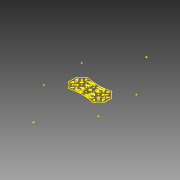
# Autodesk Inventor part: Centerplate
Saved by Autodesk Inventor 2012 (Build 160160000, 160)
## iProperties
Created: 2014-07-01
Part Number: Centerplate
Material: Default
Document SubType Name: Modeling
Designer: Laurent
Density: 1 g/cm^3
Author: Laurent
Autodesk Inventor part; units mm, degrees
ref_plane "YZ Plane" through (0, 0, 0) normal (1, 0, 0) x (0, 1, 0)
ref_plane "XZ Plane" through (0, 0, 0) normal (0, 1, 0) x (-1, 0, 0)
ref_plane "XY Plane" through (0, 0, 0) normal (0, 0, 1) x (1, 0, 0)
sketch "Sketch1" plane through (0, 0, 0) normal (0, 0, 1) x (1, 0, 0)
  line L0 (-75, 40) -> (75, 40)
  line L1 (75, 40) -> (75, -40)
  line L2 (75, -40) -> (-75, -40)
  line L3 (-75, -40) -> (-75, 40)
  point P0 (0, 0)
  dimension "d0" = 150
  dimension "d1" = 80
  dimension "d2" = 40
  dimension "d3" = 75
  constraints: 8 end point, 2 parallel, 1 horizontal, 1 perpendicular
  measures "d0" distance of L1.end L2.end
  measures "d1" distance of L0.end L1.end
  measures "d2" distance from line of L0 point (0, 0)
  measures "d3" distance from line of L1 point (0, 0)
extrude "Vlak" add sketch "Sketch1" along normal blind 4
sketch "Sketch3" plane through (0, 0, 4) normal (0, 0, 1) x (1, 0, 0)
  line L0 (75, 40) -> (75, -40) projected
  line L1 (-75, 40) -> (75, 40) projected
  circle A0 centre (75, 40) radius 10
  point P0 (0, 0)
  dimension "d12" = 20
  dimension "d13" = 0
  dimension "d14" = 0
  constraints: 1 centre point
  measures "d12" diameter of A0
  measures "d13" distance from line of L0 A0.centre
  measures "d14" distance from line of L1 A0.centre
extrude "Centergat" cut sketch "Sketch3" against normal blind 4
sketch "Sketch4" plane through (0, 0, 4) normal (0, 0, 1) x (1, 0, 0)
  line L0 (-75, 40) -> (65, 40) projected
  line L1 (75, -40) -> (-75, -40) projected
  line L2 (18.8539, 53.8539) -> (-131.8943, -96.8943) construction
  circle A0 centre (-155, -120) radius 150
  point P0 (0, 0)
  dimension "d17" = 0
  dimension "d18" = 45
  dimension "d19" = 300
  dimension "d20" = 0
  dimension "d21" = 160
  constraints: 2 end point, 1 centre point
  measures "d17" distance from line of L1.end L2
  measures "d18" angle of L1 L2
  measures "d19" diameter of A0
  measures "d20" distance from line of L2 A0.centre
  measures "d21" distance from line of L0 A0.centre
extrude "PropellorSpace" cut sketch "Sketch4" against normal blind 4
sketch "Sketch5" plane through (0, 0, 4) normal (0, 0, 1) x (1, 0, 0)
  arc A0 (-28.1142, -40) -> (-75, 6.8858) centre (-155, -120) ccw projected
  line L0 (75, -40) -> (-28.1142, -40) projected
  line L1 (-75, 40) -> (65, 40) projected
  line L2 (-155, -120) -> (34.1296, 69.1296) construction
  line L3 (-168.3606, -98.0053) -> (-8.8118, 61.5435) construction
  line L4 (-132.6124, -132.9677) -> (63.849, 63.4937) construction
  line L5 (-208.1378, -57.7825) -> (-104.1378, -161.7825) construction
  line L6 (-25.5995, -23.1264) -> (-11.4573, -8.9842)
  line L7 (-11.4573, -8.9842) -> (-8.6289, -11.8127)
  line L8 (-8.6289, -11.8127) -> (-22.771, -25.9548)
  line L9 (-22.771, -25.9548) -> (-25.5995, -23.1264)
  line L10 (-60.9548, 12.229) -> (-46.8127, 26.3711)
  line L11 (-46.8127, 26.3711) -> (-43.9842, 23.5427)
  line L12 (-43.9842, 23.5427) -> (-58.1264, 9.4005)
  line L13 (-58.1264, 9.4005) -> (-60.9548, 12.229)
  line L14 (13.2914, 15.7645) -> (27.4335, 29.9066)
  line L15 (27.4335, 29.9066) -> (30.262, 27.0782)
  line L16 (30.262, 27.0782) -> (16.1198, 12.9361)
  line L17 (16.1198, 12.9361) -> (13.2914, 15.7645)
  line L18 (-62.0184, 71.663) -> (40.1093, -30.4647) construction
  line L19 (-7.9217, 14.7379) -> (-22.0638, 28.88)
  line L20 (-22.0638, 28.88) -> (-19.2354, 31.7085)
  line L21 (-19.2354, 31.7085) -> (-5.0932, 17.5663)
  line L22 (-5.0932, 17.5663) -> (-7.9217, 14.7379)
  point P0 (0, 0)
  point P1 (-168.1378, -97.7825)
  point P2 (-132.7825, -133.1378)
  point P3 (-30.3553, 40)
  dimension "d24" = 45
  dimension "d25" = 0
  dimension "d26" = 90
  dimension "d27" = 25
  dimension "d28" = 25
  dimension "d29" = 0
  dimension "d30" = 0
  dimension "d31" = 0
  dimension "d32" = 20
  dimension "d33" = 4
  dimension "d34" = 20
  dimension "d35" = 4
  dimension "d36" = 0
  dimension "d37" = 2
  dimension "d38" = 0
  dimension "d39" = 2
  dimension "d40" = 160
  dimension "d41" = 160
  dimension "d44" = 55
  dimension "d49" = 45
  dimension "d50" = 0
  dimension "d51" = 0
  dimension "d52" = 0
  dimension "d53" = 21.2742
  dimension "d54" = 20
  dimension "d55" = 4
  dimension "d56" = 0
  dimension "d57" = 2
  dimension "d58" = 13.726
  constraints: 42 end point, 6 parallel, 4 perpendicular, 2 point on line, 1 collinear, 8 other
  measures "d24" angle of L0 L2
  measures "d25" angle of L3 L2
  measures "d26" angle of L2 L5
  measures "d27" distance from line of L2 point (-168.138, -97.783)
  measures "d28" distance from line of L2 point (-132.783, -133.138)
  measures "d29" distance from line of point (-132.783, -133.138) L4
  measures "d30" distance from line of point (-168.138, -97.783) L3
  measures "d31" angle of L4 L2
  measures "d32" distance of L7.end L8.end
  measures "d33" distance of L6.end L7.end
  measures "d34" distance of L11.end L13.start
  measures "d35" distance of L10.end L11.end
  measures "d36" angle of L3 L10
  measures "d37" distance from line of L3 L10.end
  measures "d38" angle of L4 L6
  measures "d39" distance from line of L4 L7.end
  measures "d40" distance from line of L2.start L13
  measures "d41" distance from line of L2.start L9
  measures "d44" distance of L7.end L16.start
  measures "d49" angle of L1 L18
  measures "d50" distance from line of L3 point (-30.355, 40)
  measures "d51" distance from line of L1 point (-30.355, 40)
  measures "d52" distance from line of point (-30.355, 40) L18
  measures "d53" distance from line of point (-30.355, 40) L11
  measures "d54" distance of L20.end L21.end
  measures "d55" distance of L19.end L20.end
  measures "d56" angle of L18 L19
  measures "d57" distance from line of L18 L20.end
  measures "d58" distance from line of L20 point (-30.355, 40)
extrude "Armsteunen" cut sketch "Sketch5" against normal blind 4
sketch "Sketch6" plane through (0, 0, 4) normal (0, 0, 1) x (1, 0, 0)
  line L0 (75, -40) -> (-28.1142, -40) projected
  line L1 (75, 30) -> (75, -40) projected
  line L2 (-75, 40) -> (65, 40) projected
  line L3 (-75, 6.8858) -> (-75, 40) projected
  circle A0 centre (55, -20) radius 1.5
  circle A1 centre (15, -20) radius 1.5
  circle A2 centre (-13.9878, -20) radius 1.5
  circle A3 centre (-34.4939, 0.5061) radius 1.5
  circle A4 centre (43.89, 40) radius 1.5
  circle A5 centre (26.0122, 20) radius 1.5
  circle A6 centre (5, 40) radius 1.5
  circle A7 centre (-55, 21.0122) radius 1.5
  circle A8 centre (-55, 30) radius 1.5
  line L4 (-55, 21.0122) -> (-13.9878, -20) construction
  line L5 (-34.4939, 0.5061) -> (12.7873, 47.7873) construction
  circle A9 centre (-40.4428, 35) radius 1.5
  circle A10 centre (3.6899, -2.3223) radius 1.5
  circle A11 centre (-16.8162, 18.1838) radius 1.5
  arc A12 (65, 40) -> (75, 30) centre (75, 40) ccw projected
  circle A13 centre (75, 8.89) radius 1.5
  point P0 (0, 0)
  point P1 (-43.9842, 23.5427)
  point P2 (-11.4573, -8.9842)
  dimension "d61" = 3
  dimension "d62" = 3
  dimension "d63" = 3
  dimension "d64" = 3
  dimension "d65" = 3
  dimension "d66" = 3
  dimension "d67" = 3
  dimension "d68" = 3
  dimension "d69" = 3
  dimension "d70" = 20
  dimension "d71" = 20
  dimension "d72" = 20
  dimension "d73" = 60
  dimension "d75" = 20
  dimension "d76" = 31.11
  dimension "d77" = 0
  dimension "d78" = 20
  dimension "d80" = 10
  dimension "d82" = 20
  dimension "d83" = 20
  dimension "d84" = 0
  dimension "d87" = 45
  dimension "d88" = 0
  dimension "d89" = 0
  dimension "d90" = 3
  dimension "d101" = 3
  dimension "d103" = 29
  dimension "d106" = 3
  dimension "d107" = 0
  dimension "d111" = 3
  dimension "d112" = 0
  dimension "d113" = 31.11
  dimension "d166" = 29
  dimension "d167" = 23
  dimension "d168" = 23
  dimension "d169" = 29
  dimension "d170" = 25
  dimension "d171" = 25
  dimension "d172" = 29
  dimension "d175" = 29
  dimension "d179" = 5
  dimension "d182" = 43.9962
  constraints: 13 centre point, 4 end point
  measures "d61" diameter of A0
  measures "d62" diameter of A1
  measures "d63" diameter of A2
  measures "d64" diameter of A3
  measures "d65" diameter of A4
  measures "d66" diameter of A5
  measures "d67" diameter of A6
  measures "d68" diameter of A7
  measures "d69" diameter of A8
  measures "d70" distance from line of L1 A0.centre
  measures "d71" distance from line of L0 A0.centre
  measures "d72" distance from line of L0 A1.centre
  measures "d73" distance from line of L1 A1.centre
  measures "d75" distance from line of L0 L4.end
  measures "d76" distance from line of L1 A4.centre
  measures "d77" distance from line of L2 A4.centre
  measures "d78" distance from line of L2 A5.centre
  measures "d80" distance from line of L2 A8.centre
  measures "d82" distance from line of L3 L4.start
  measures "d83" distance from line of L3 A8.centre
  measures "d84" distance from line of L4 L5.start
  measures "d87" angle of L2 L5
  measures "d88" distance from line of L2 A6.centre
  measures "d89" distance from line of L5 A6.centre
  measures "d90" diameter of A9
  measures "d101" diameter of A10
  measures "d103" distance from line of A10.centre L5
  measures "d106" diameter of A11
  measures "d107" distance from line of L5 A11.centre
  measures "d111" diameter of A13
  measures "d112" distance from line of L1 A13.centre
  measures "d113" distance of A12.centre A13.centre
  measures "d166" distance from line of L4.end L5
  measures "d167" distance from line of point (-11.457, -8.984) L5
  measures "d168" distance from line of point (-43.984, 23.543) L5
  measures "d169" distance from line of L4.start L5
  measures "d170" distance of A11.centre L5.start
  measures "d171" distance of A10.centre L4.end
  measures "d172" distance of A9.centre A11.centre
  measures "d175" distance from line of L5 A5.centre
  measures "d179" distance from line of A9.centre L2
  measures "d182" distance of A13.centre A4.centre
extrude "Holes" cut sketch "Sketch6" against normal blind 4
sketch "Sketch10" plane through (0, 0, 4) normal (0, 0, 1) x (1, 0, 0)
  line L0 (45.39, 40) -> (65, 40) projected
  line L1 (6.5, 40) -> (42.39, 40) projected
  line L2 (75, 7.39) -> (75, -40) projected
  line L3 (45, -8) -> (65, -8)
  line L4 (65, -8) -> (65, -12)
  line L5 (65, -12) -> (45, -12)
  line L6 (45, -12) -> (45, -8)
  line L7 (31, 30) -> (35, 30)
  line L8 (35, 30) -> (35, 10)
  line L9 (35, 10) -> (31, 10)
  line L10 (31, 10) -> (31, 30)
  line L11 (5, -8) -> (25, -8)
  line L12 (25, -8) -> (25, -12)
  line L13 (25, -12) -> (5, -12)
  line L14 (5, -12) -> (5, -8)
  point P0 (0, 0)
  point P1 (-8.6289, -11.8127)
  dimension "d114" = 20
  dimension "d115" = 4
  dimension "d116" = 4
  dimension "d117" = 20
  dimension "d118" = 10
  dimension "d119" = 48
  dimension "d120" = 40
  dimension "d121" = 10
  dimension "d124" = 40
  dimension "d164" = 13.6289
  dimension "d165" = 10
  constraints: 24 end point, 4 parallel, 3 horizontal, 2 perpendicular, 1 collinear, 7 other
  measures "d114" distance of L4.end L5.end
  measures "d115" distance of L3.end L4.end
  measures "d116" distance of L8.end L9.end
  measures "d117" distance of L7.end L8.end
  measures "d118" distance from line of L2 L4.end
  measures "d119" distance between parallel lines of L0 L3
  measures "d120" distance between parallel lines of L2 L8
  measures "d121" distance between parallel lines of L1 L7
  measures "d124" distance of L3.start L14.end
  measures "d164" distance from line of L14 point (-8.629, -11.813)
  measures "d165" distance between parallel lines of L6 L8
extrude "InternalStructure" cut sketch "Sketch10" against normal blind 4
sketch "Sketch11" plane through (0, 0, 4) normal (0, 0, 1) x (1, 0, 0)
  line L0 (25, -8) -> (25, -12) projected
  line L1 (-25.5995, -23.1264) -> (-11.4573, -8.9842) projected
  circle A0 centre (15, -20) radius 1.5 projected
  circle A1 centre (-34.4939, 0.5061) radius 1.5 projected
  line L2 (6.5, 40) -> (42.39, 40) projected
  line L3 (75, 7.39) -> (75, -40) projected
  line L4 (40, 25) -> (50, 25)
  line L5 (50, 25) -> (50, 0)
  line L6 (50, 0) -> (40, 0)
  line L7 (40, 0) -> (40, 25)
  line L8 (25, -15) -> (45, -15)
  line L9 (45, -15) -> (45, -25)
  line L10 (45, -25) -> (25, -25)
  line L11 (25, -25) -> (25, -15)
  line L12 (-24.6985, 17.3726) -> (-17.6274, 10.3015)
  line L13 (-17.6274, 10.3015) -> (-28.234, -0.3051)
  line L14 (-28.234, -0.3051) -> (-35.3051, 6.766)
  line L15 (-35.3051, 6.766) -> (-24.6985, 17.3726)
  line L16 (-7.9217, 14.7379) -> (-22.0638, 28.88) projected
  point P0 (0, 0)
  dimension "d134" = 10
  dimension "d135" = 25
  dimension "d136" = 25
  dimension "d137" = 15
  dimension "d138" = 20
  dimension "d139" = 10
  dimension "d140" = 0
  dimension "d141" = 5
  dimension "d142" = 10
  dimension "d144" = 0
  dimension "d145" = 5
  dimension "d180" = 10
  dimension "d181" = 15
  constraints: 24 end point, 6 parallel, 3 perpendicular, 2 horizontal
  measures "d134" distance of L5.end L6.end
  measures "d135" distance of L4.end L5.end
  measures "d136" distance between parallel lines of L3 L5
  measures "d137" distance between parallel lines of L2 L4
  measures "d138" distance of L9.end L10.end
  measures "d139" distance of L8.end L9.end
  measures "d140" distance between parallel lines of L0 L11
  measures "d141" distance from line of L8 A0.centre
  measures "d142" distance of L13.end L14.end
  measures "d144" angle of L1 L13
  measures "d145" distance from line of A1.centre L13
  measures "d180" distance from line of L16 L12.start
  measures "d181" distance between parallel lines of L12 L14
extrude "CablingHoles" cut sketch "Sketch11" against normal blind 4 contours L4 L5 L6 L7 | L8 L9 L10 L11 | L12 L13 L14 L15
sketch "Sketch12" plane through (0, 0, 4) normal (0, 0, 1) x (1, 0, 0)
  line L0 (75, -40) -> (-28.1142, -40) projected
  line L1 (75, 7.39) -> (75, -40) projected
  arc A0 (75, -26.5) -> (-28.1142, -40) centre (76.1332, -435.7032) ccw
  line L2 (45, -25) -> (25, -25) projected
  line L3 (5, -8) -> (25, -8) projected
  line L4 (35, 30) -> (35, -49) construction
  line L5 (65, -8) -> (-10, -8) construction
  circle A1 centre (29, -5) radius 1.5
  circle A2 centre (38, -5) radius 1.5
  line L6 (16.1198, 12.9361) -> (13.2914, 15.7645) projected
  line L7 (-7.9217, 14.7379) -> (-22.0638, 28.88) projected
  line L8 (-22.0638, 28.88) -> (-19.2354, 31.7085) projected
  line L9 (-19.2354, 31.7085) -> (-5.0932, 17.5663) projected
  line L10 (-46.8127, 26.3711) -> (-43.9842, 23.5427) projected
  line L11 (-43.9842, 23.5427) -> (-58.1264, 9.4005) projected
  point P0 (0, 0)
  dimension "d149" = 13.5
  dimension "d150" = 103.1142
  dimension "d151" = 40
  dimension "d156" = 3
  dimension "d157" = 3
  dimension "d158" = 3
  dimension "d159" = 3
  dimension "d160" = 6
  dimension "d161" = 3
  dimension "d176" = 11.7258
  dimension "d177" = 11.726
  dimension "d178" = 19.2742
  constraints: 4 end point, 3 centre point, 2 point on circle, 2 point on line, 1 perpendicular
  measures "d149" distance of L0.start A0.start
  measures "d150" distance from line of L1 L0.end
  measures "d151" vertical distance of point (0, 0) L0.end
  measures "d156" diameter of A1
  measures "d157" diameter of A2
  measures "d158" distance from line of L5 A2.centre
  measures "d159" distance from line of L4 A2.centre
  measures "d160" distance from line of L4 A1.centre
  measures "d161" distance from line of L5 A1.centre
  measures "d176" distance between parallel lines of L6 L9
  measures "d177" distance between parallel lines of L8 L11
  measures "d178" distance between parallel lines of L7 L10
extrude "BodyReshape" cut sketch "Sketch12" against normal blind 4
sketch "Sketch14" plane through (0, 0, 4) normal (0, 0, 1) x (1, 0, 0)
  arc A0 (75, -26.5) -> (-28.1142, -40) centre (76.1332, -435.7032) ccw projected
  line L0 (75, 7.39) -> (75, -26.5) projected
  arc A1 (75, 10.39) -> (75, 7.39) centre (75, 8.89) ccw projected
  line L1 (75, 30) -> (75, 10.39) projected
  arc A2 (65, 40) -> (75, 30) centre (75, 40) ccw projected
  line L2 (45.39, 40) -> (65, 40) projected
  arc A3 (42.39, 40) -> (45.39, 40) centre (43.89, 40) ccw projected
  line L3 (6.5, 40) -> (42.39, 40) projected
  arc A4 (3.5, 40) -> (6.5, 40) centre (5, 40) ccw projected
  line L4 (-75, 40) -> (3.5, 40) projected
  arc A5 (-28.1142, -40) -> (-75, 6.8858) centre (-155, -120) ccw projected
  circle A6 centre (-55, 21.0122) radius 1.5 projected
  circle A7 centre (-34.4939, 0.5061) radius 1.5 projected
  circle A8 centre (-13.9878, -20) radius 1.5 projected
  circle A9 centre (55, -20) radius 1.5 projected
  circle A10 centre (-16.8162, 18.1838) radius 1.5 projected
  circle A11 centre (3.6899, -2.3223) radius 1.5 projected
  circle A12 centre (-55, 30) radius 1.5 projected
  circle A13 centre (15, -20) radius 1.5 projected
  circle A14 centre (26.0122, 20) radius 1.5 projected
  circle A15 centre (-40.4428, 35) radius 1.5 projected
  circle A16 centre (29, -5) radius 1.5 projected
  circle A17 centre (38, -5) radius 1.5 projected
  arc A18 (178.1142, -40) -> (75, -26.5) centre (73.8668, -435.7032) ccw
  arc A19 (75, 7.39) -> (75, 10.39) centre (75, 8.89) ccw
  arc A20 (75, 30) -> (85, 40) centre (75, 40) ccw
  line L5 (104.61, 40) -> (85, 40)
  arc A21 (104.61, 40) -> (107.61, 40) centre (106.11, 40) ccw
  line L6 (143.5, 40) -> (107.61, 40)
  arc A22 (143.5, 40) -> (146.5, 40) centre (145, 40) ccw
  line L7 (225, 40) -> (146.5, 40)
  line L8 (225, 6.8858) -> (225, 40)
  arc A23 (225, 6.8858) -> (178.1142, -40) centre (305, -120) ccw
  circle A24 centre (205, 21.0122) radius 1.5
  circle A25 centre (184.4939, 0.5061) radius 1.5
  circle A26 centre (163.9878, -20) radius 1.5
  circle A27 centre (95, -20) radius 1.5
  circle A28 centre (166.8162, 18.1838) radius 1.5
  circle A29 centre (146.3101, -2.3223) radius 1.5
  circle A30 centre (205, 30) radius 1.5
  circle A31 centre (135, -20) radius 1.5
  circle A32 centre (123.9878, 20) radius 1.5
  circle A33 centre (190.4428, 35) radius 1.5
  line L9 (208.1264, 9.4005) -> (210.9548, 12.229)
  line L10 (210.9548, 12.229) -> (196.8127, 26.3711)
  line L11 (196.8127, 26.3711) -> (193.9842, 23.5427)
  line L12 (193.9842, 23.5427) -> (208.1264, 9.4005)
  line L13 (155.0932, 17.5663) -> (157.9217, 14.7379)
  line L14 (157.9217, 14.7379) -> (172.0638, 28.88)
  line L15 (172.0638, 28.88) -> (169.2354, 31.7085)
  line L16 (169.2354, 31.7085) -> (155.0932, 17.5663)
  line L17 (172.771, -25.9548) -> (175.5995, -23.1264)
  line L18 (175.5995, -23.1264) -> (161.4573, -8.9842)
  line L19 (161.4573, -8.9842) -> (158.6289, -11.8127)
  line L20 (158.6289, -11.8127) -> (172.771, -25.9548)
  line L21 (136.7086, 15.7645) -> (122.5665, 29.9066)
  line L22 (122.5665, 29.9066) -> (119.738, 27.0782)
  line L23 (119.738, 27.0782) -> (133.8802, 12.9361)
  line L24 (133.8802, 12.9361) -> (136.7086, 15.7645)
  line L25 (105, -12) -> (105, -8)
  line L26 (105, -8) -> (85, -8)
  line L27 (85, -8) -> (85, -12)
  line L28 (85, -12) -> (105, -12)
  line L29 (145, -12) -> (145, -8)
  line L30 (145, -8) -> (125, -8)
  line L31 (125, -8) -> (125, -12)
  line L32 (125, -12) -> (145, -12)
  line L33 (119, 10) -> (119, 30)
  line L34 (119, 30) -> (115, 30)
  line L35 (115, 30) -> (115, 10)
  line L36 (115, 10) -> (119, 10)
  line L37 (185.3051, 6.766) -> (174.6985, 17.3726)
  line L38 (174.6985, 17.3726) -> (167.6274, 10.3015)
  line L39 (167.6274, 10.3015) -> (178.234, -0.3051)
  line L40 (178.234, -0.3051) -> (185.3051, 6.766)
  line L41 (110, 0) -> (110, 25)
  line L42 (110, 25) -> (100, 25)
  line L43 (100, 25) -> (100, 0)
  line L44 (100, 0) -> (110, 0)
  line L45 (125, -25) -> (125, -15)
  line L46 (125, -15) -> (105, -15)
  line L47 (105, -15) -> (105, -25)
  line L48 (105, -25) -> (125, -25)
  circle A34 centre (121, -5) radius 1.5
  circle A35 centre (112, -5) radius 1.5
  arc A36 (-28.1142, 120) -> (75, 106.5) centre (76.1332, 515.7032) ccw
  line L49 (75, 72.61) -> (75, 106.5)
  arc A37 (75, 72.61) -> (75, 69.61) centre (75, 71.11) ccw
  line L50 (75, 50) -> (75, 69.61)
  arc A38 (75, 50) -> (65, 40) centre (75, 40) ccw
  arc A39 (45.39, 40) -> (42.39, 40) centre (43.89, 40) ccw
  arc A40 (6.5, 40) -> (3.5, 40) centre (5, 40) ccw
  line L51 (-75, 73.1142) -> (-75, 40)
  arc A41 (-75, 73.1142) -> (-28.1142, 120) centre (-155, 200) ccw
  circle A42 centre (-55, 58.9878) radius 1.5
  circle A43 centre (-34.4939, 79.4939) radius 1.5
  circle A44 centre (-13.9878, 100) radius 1.5
  circle A45 centre (55, 100) radius 1.5
  circle A46 centre (-16.8162, 61.8162) radius 1.5
  circle A47 centre (3.6899, 82.3223) radius 1.5
  circle A48 centre (-55, 50) radius 1.5
  circle A49 centre (15, 100) radius 1.5
  circle A50 centre (26.0122, 60) radius 1.5
  circle A51 centre (-40.4428, 45) radius 1.5
  line L52 (-58.1264, 70.5995) -> (-60.9548, 67.771)
  line L53 (-60.9548, 67.771) -> (-46.8127, 53.6289)
  line L54 (-46.8127, 53.6289) -> (-43.9842, 56.4573)
  line L55 (-43.9842, 56.4573) -> (-58.1264, 70.5995)
  line L56 (-5.0932, 62.4337) -> (-7.9217, 65.2621)
  line L57 (-7.9217, 65.2621) -> (-22.0638, 51.12)
  line L58 (-22.0638, 51.12) -> (-19.2354, 48.2915)
  line L59 (-19.2354, 48.2915) -> (-5.0932, 62.4337)
  line L60 (-22.771, 105.9548) -> (-25.5995, 103.1264)
  line L61 (-25.5995, 103.1264) -> (-11.4573, 88.9842)
  line L62 (-11.4573, 88.9842) -> (-8.6289, 91.8127)
  line L63 (-8.6289, 91.8127) -> (-22.771, 105.9548)
  line L64 (13.2914, 64.2355) -> (27.4335, 50.0934)
  line L65 (27.4335, 50.0934) -> (30.262, 52.9218)
  line L66 (30.262, 52.9218) -> (16.1198, 67.0639)
  line L67 (16.1198, 67.0639) -> (13.2914, 64.2355)
  line L68 (45, 92) -> (45, 88)
  line L69 (45, 88) -> (65, 88)
  line L70 (65, 88) -> (65, 92)
  line L71 (65, 92) -> (45, 92)
  line L72 (5, 92) -> (5, 88)
  line L73 (5, 88) -> (25, 88)
  line L74 (25, 88) -> (25, 92)
  line L75 (25, 92) -> (5, 92)
  line L76 (31, 70) -> (31, 50)
  line L77 (31, 50) -> (35, 50)
  line L78 (35, 50) -> (35, 70)
  line L79 (35, 70) -> (31, 70)
  line L80 (-35.3051, 73.234) -> (-24.6985, 62.6274)
  line L81 (-24.6985, 62.6274) -> (-17.6274, 69.6985)
  line L82 (-17.6274, 69.6985) -> (-28.234, 80.3051)
  line L83 (-28.234, 80.3051) -> (-35.3051, 73.234)
  line L84 (40, 80) -> (40, 55)
  line L85 (40, 55) -> (50, 55)
  line L86 (50, 55) -> (50, 80)
  line L87 (50, 80) -> (40, 80)
  line L88 (25, 105) -> (25, 95)
  line L89 (25, 95) -> (45, 95)
  line L90 (45, 95) -> (45, 105)
  line L91 (45, 105) -> (25, 105)
  circle A52 centre (29, 85) radius 1.5
  circle A53 centre (38, 85) radius 1.5
  line L92 (100, 80) -> (110, 80)
  line L93 (115, 70) -> (119, 70)
  line L94 (100, 55) -> (100, 80)
  line L95 (110, 55) -> (100, 55)
  line L96 (119, 70) -> (119, 50)
  line L97 (119, 50) -> (115, 50)
  line L98 (115, 50) -> (115, 70)
  arc A54 (75, 69.61) -> (75, 72.61) centre (75, 71.11) ccw
  arc A55 (85, 40) -> (75, 50) centre (75, 40) ccw
  line L99 (110, 80) -> (110, 55)
  line L100 (178.234, 80.3051) -> (185.3051, 73.234)
  line L101 (167.6274, 69.6985) -> (178.234, 80.3051)
  arc A56 (178.1142, 120) -> (225, 73.1142) centre (305, 200) ccw
  circle A57 centre (184.4939, 79.4939) radius 1.5
  line L102 (161.4573, 88.9842) -> (158.6289, 91.8127)
  line L103 (175.5995, 103.1264) -> (161.4573, 88.9842)
  line L104 (158.6289, 91.8127) -> (172.771, 105.9548)
  line L105 (172.771, 105.9548) -> (175.5995, 103.1264)
  circle A58 centre (163.9878, 100) radius 1.5
  line L106 (105, 88) -> (85, 88)
  line L107 (85, 88) -> (85, 92)
  line L108 (85, 92) -> (105, 92)
  circle A59 centre (95, 100) radius 1.5
  line L109 (174.6985, 62.6274) -> (167.6274, 69.6985)
  line L110 (185.3051, 73.234) -> (174.6985, 62.6274)
  circle A60 centre (166.8162, 61.8162) radius 1.5
  line L111 (208.1264, 70.5995) -> (210.9548, 67.771)
  line L112 (196.8127, 53.6289) -> (193.9842, 56.4573)
  line L113 (193.9842, 56.4573) -> (208.1264, 70.5995)
  circle A61 centre (205, 58.9878) radius 1.5
  line L114 (210.9548, 67.771) -> (196.8127, 53.6289)
  circle A62 centre (190.4428, 45) radius 1.5
  line L115 (155.0932, 62.4337) -> (157.9217, 65.2621)
  line L116 (172.0638, 51.12) -> (169.2354, 48.2915)
  line L117 (157.9217, 65.2621) -> (172.0638, 51.12)
  line L118 (169.2354, 48.2915) -> (155.0932, 62.4337)
  circle A63 centre (205, 50) radius 1.5
  line L119 (225, 73.1142) -> (225, 40)
  circle A64 centre (112, 85) radius 1.5
  line L120 (105, 92) -> (105, 88)
  circle A65 centre (121, 85) radius 1.5
  line L121 (125, 88) -> (125, 92)
  line L122 (125, 95) -> (105, 95)
  line L123 (105, 95) -> (105, 105)
  line L124 (125, 105) -> (125, 95)
  line L125 (105, 105) -> (125, 105)
  arc A66 (75, 106.5) -> (178.1142, 120) centre (73.8668, 515.7032) ccw
  arc A67 (107.61, 40) -> (104.61, 40) centre (106.11, 40) ccw
  arc A68 (146.5, 40) -> (143.5, 40) centre (145, 40) ccw
  line L126 (133.8802, 67.0639) -> (136.7086, 64.2355)
  line L127 (136.7086, 64.2355) -> (122.5665, 50.0934)
  line L128 (122.5665, 50.0934) -> (119.738, 52.9218)
  line L129 (119.738, 52.9218) -> (133.8802, 67.0639)
  circle A69 centre (123.9878, 60) radius 1.5
  line L130 (145, 92) -> (145, 88)
  line L131 (145, 88) -> (125, 88)
  line L132 (125, 92) -> (145, 92)
  circle A70 centre (135, 100) radius 1.5
  circle A71 centre (146.3101, 82.3223) radius 1.5
  point P0 (-58.1264, 9.4005)
  point P1 (-60.9548, 12.229)
  point P2 (-46.8127, 26.3711)
  point P3 (-43.9842, 23.5427)
  point P4 (-5.0932, 17.5663)
  point P5 (-7.9217, 14.7379)
  point P6 (-22.0638, 28.88)
  point P7 (-19.2354, 31.7085)
  point P8 (-22.771, -25.9548)
  point P9 (-25.5995, -23.1264)
  point P10 (-11.4573, -8.9842)
  point P11 (-8.6289, -11.8127)
  point P12 (13.2914, 15.7645)
  point P13 (27.4335, 29.9066)
  point P14 (30.262, 27.0782)
  point P15 (16.1198, 12.9361)
  point P16 (45, -12)
  point P17 (45, -8)
  point P18 (65, -8)
  point P19 (65, -12)
  point P20 (5, -12)
  point P21 (5, -8)
  point P22 (25, -8)
  point P23 (25, -12)
  point P24 (31, 10)
  point P25 (31, 30)
  point P26 (35, 30)
  point P27 (35, 10)
  point P28 (-35.3051, 6.766)
  point P29 (-24.6985, 17.3726)
  point P30 (-17.6274, 10.3015)
  point P31 (-28.234, -0.3051)
  point P32 (40, 0)
  point P33 (40, 25)
  point P34 (50, 25)
  point P35 (50, 0)
  point P36 (25, -25)
  point P37 (25, -15)
  point P38 (45, -15)
  point P39 (45, -25)
  point P40 (0, 0)
  point P41 (150, 0)
  point P42 (0, 80)
  point P43 (150, 80)
  constraints: 256 end point, 184 symmetric about line, 54 centre point, 36 point on circle, 54 other
extrude "Mirroring" add sketch "Sketch14" against normal blind 4 contours A19 L1 A20 L5 A21 L6 A22 L7 L8 A23 A18 L0 | L2 A39 L3 A40 L4 L51 A41 A36 L49 A37 L50 A38 | A55 L50 A54 L49 A66 A56 L119 L7 A68 L6 A67 L5
body "Solid2"
